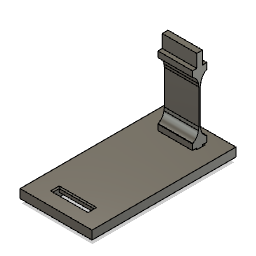
flexure thin v2 (Autodesk Fusion 360 design; units mm, degrees)
Autodesk Fusion 360 part; units mm, degrees
sketch "Sketch1" plane through (0, 0, 0) normal (1, 0, 0) x (0, 0, -1)
  line L0 (0, 0) -> (2, 0)
  line L1 (2, 0) -> (2, -4.5)
  line L2 (2, -4.5) -> (0, -4.5)
  line L3 (0, -4.5) -> (0, 0)
  line L4 (2, 0) -> (3.5, 0)
  line L5 (1, 0) -> (1, 16.3106) construction
  line L6 (-3.4591, 11.9915) -> (5.8046, 11.9915) construction
  line L7 (1.25, 11.9915) -> (1.25, 5.9915)
  line L8 (1.25, 5.9915) -> (1.7, 3.0254)
  line L9 (3.5, 0) -> (3.5, 2)
  line L10 (3.5, 2) -> (1.7, 3.0254)
  line L11 (0, 0) -> (-1.5, 0)
  line L12 (-1.5, 0) -> (-1.5, 2)
  line L13 (-1.5, 2) -> (0.3, 3.0254)
  line L14 (0.75, 5.9915) -> (0.3, 3.0254)
  line L15 (0.75, 11.9915) -> (0.75, 5.9915)
  line L16 (2, 23.9829) -> (3.5, 23.9829)
  line L17 (0.75, 17.9915) -> (0.3, 20.9575)
  line L18 (1.25, 17.9915) -> (1.7, 20.9575)
  line L19 (0.75, 11.9915) -> (0.75, 17.9915)
  line L20 (3.5, 23.9829) -> (3.5, 21.9829)
  line L21 (1.25, 11.9915) -> (1.25, 17.9915)
  line L22 (2, 23.9829) -> (2, 28.4829)
  line L23 (-1.5, 21.9829) -> (0.3, 20.9575)
  line L24 (0, 28.4829) -> (0, 23.9829)
  line L25 (2, 28.4829) -> (0, 28.4829)
  line L26 (0, 23.9829) -> (-1.5, 23.9829)
  line L27 (-1.5, 23.9829) -> (-1.5, 21.9829)
  line L28 (0, 23.9829) -> (2, 23.9829)
  line L29 (3.5, 21.9829) -> (1.7, 20.9575)
  point P0 (0, 23.9829)
  point P1 (1, 23.9829)
  dimension "d1" = 2
  dimension "d2" = 4.5
  dimension "d3" = 1.5
  dimension "d6" = 6
  dimension "d7" = 3
  dimension "d8" = 0.25
  dimension "d9" = 0.7
  dimension "d10" = 2
  dimension "d24" = 1.0254
  constraint horizontal L0
  constraint vertical L1
  constraint horizontal L2
  constraint vertical L3
  constraint coincident L0.start L3.end
  constraint perpendicular L1 L4
  constraint midpoint L0 L5.start
  constraint perpendicular L0 L5
  constraint horizontal L6
  constraint coincident L6 L7.start
  constraint perpendicular L6 L7
  constraint perpendicular L4 L9
  constraint symmetric L0.end L5 L0.start
  constraint symmetric L4.end L5 L11.end
  constraint symmetric L5 L7.start L15.start
  constraint symmetric L5 L7.end L14.start
  constraint symmetric L5 L8.end L13.end
  constraint symmetric L5 L9.end L12.end
  constraint symmetric L0.start L6 L24.end
  constraint symmetric L0.start L6 P0
  constraint symmetric L0.end L6 L16.start
  constraint symmetric L1.end L6 L22.end
  constraint symmetric L2.end L6 L24.start
  constraint symmetric L4.end L6 L16.end
  constraint symmetric L5.start L6 P1
  constraint symmetric L6 L7.start L21.start
  constraint symmetric L6 L7.end L18.start
  constraint symmetric L6 L8.end L18.end
  constraint symmetric L6 L9.end L20.end
  constraint symmetric L6 L0.start P0
  constraint symmetric L6 L11.end L26.end
  constraint symmetric L6 L12.end L23.start
  constraint symmetric L6 L13.end L17.end
  constraint symmetric L6 L14.start L17.start
  constraint symmetric L6 L15.start L19.start
  measures "d1" distance of L0.start L0.end
  measures "d2" distance of L0.start L2.end
  measures "d3" distance of L0.end L4.end
  measures "d6" distance of L7.start L7.end
  measures "d7" distance of L7.end L8.end
  measures "d8" distance of L5 L7
  measures "d9" distance of L5 L8.end
  measures "d10" distance of L4.end L9.end
  measures "d24" vertical distance of L8.end L9.end
extrude "Extrude1" add sketch "Sketch1" along normal mid plane 12 makes body 1
sketch "Sketch2" plane through (0, 0, 0) normal (0, 1, 0) x (1, 0, 0)
  line L0 (-6, 0) -> (6, 0)
  line L1 (6, 0) -> (6, 2)
  line L2 (6, 2) -> (-6, 2)
  line L3 (-6, 2) -> (-6, 0)
  line L4 (6.1, 2.1) -> (-6.1, 2.1)
  line L5 (-6.1, 2.1) -> (-6.1, -0.1)
  line L6 (-6.1, -0.1) -> (6.1, -0.1)
  line L7 (6.1, -0.1) -> (6.1, 2.1)
  line L8 (0, 0) -> (0, -36.4952) construction
  line L9 (12.5, 7.1) -> (-12.5, 7.1)
  line L10 (-12.5, 7.1) -> (-12.5, -42.9)
  line L11 (-12.5, -42.9) -> (12.5, -42.9)
  line L12 (12.5, -42.9) -> (12.5, 7.1)
  line L13 (12.5, 7.1) -> (-12.5, -42.9) construction
  line L14 (-12.5, 7.1) -> (12.5, -42.9) construction
  line L15 (0, -17.9) -> (-15.1957, -17.9) construction
  line L16 (-6.1, -35.7) -> (6.1, -35.7)
  line L17 (6.1, -35.7) -> (6.1, -37.9)
  line L18 (6.1, -37.9) -> (-6.1, -37.9)
  line L19 (-6.1, -37.9) -> (-6.1, -35.7)
  point P0 (0, -17.9)
  dimension "d13" = 0.1
  dimension "d14" = 25
  dimension "d15" = 50
  dimension "d16" = 5
  constraint coincident L8.start origin
  constraint perpendicular L6 L8
  constraint horizontal L9
  constraint perpendicular L9 L10
  constraint parallel L9 L11
  constraint parallel L10 L12
  constraint coincident L13 P0
  constraint coincident L14 P0
  constraint coincident L8 P0
  constraint coincident P0 L15.start
  constraint perpendicular L8 L15
  constraint symmetric L4.start L15 L17.end
  constraint symmetric L4.end L15 L18.end
  constraint symmetric L5.end L15 L16.start
  constraint symmetric L6.end L15 L16.end
  measures "d14" distance of L10.end L11.end
  measures "d15" distance of L9.end L10.end
  measures "d16" distance of L4 L9
extrude "Extrude2" add sketch "Sketch2" against normal blind 3 separate body contours L9 L10 L11 L12 makes body 2
chamfer "Chamfer1" distance 1.5 angle 45 4 edges at (0, -3, -2.1) (0, -3, 0.1) (0, -3, 35.7) (0, -3, 37.9) on bodies 2
fillet "Fillet1" radius 4 4 edges at (0, 3.0254, -0.3) (0, 3.0254, -1.7) (0, 20.9575, -0.3) (0, 20.9575, -1.7) on bodies 1
chamfer "Chamfer2" distance 0.4 angle 45 8 edges at (0, 0, 37.9) (-6.1, 0, 36.8) (0, 0, 35.7) (6.1, 0, 36.8) (0, 0, 0.1) (0, 0, -2.1) (6.1, 0, -1) (-6.1, 0, -1) on bodies 2
named bodies: "flexure flex thin", "flexure plate thin"
